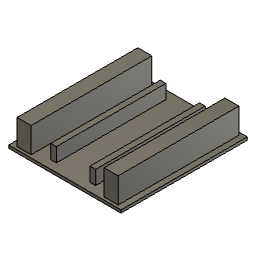
Nano Grove Shield (Autodesk Fusion 360 design; units mm, degrees)
Autodesk Fusion 360 part; units mm, degrees
sketch "Sketch1" plane through (0, 0, 0) normal (0, 1, 0) x (1, 0, 0)
  line L0 (0, 0) -> (40, 0)
  line L1 (40, 0) -> (40, -45)
  line L2 (40, -45) -> (0, -45)
  line L3 (0, -45) -> (0, 0)
  dimension "d1" = 40
  dimension "d2" = 45
  constraint horizontal L0
  constraint vertical L1
  constraint horizontal L2
  constraint vertical L3
  constraint coincident L0.start L3.end
  measures "d1" distance of L0.start L0.end
  measures "d2" distance of L0.start L2.end
extrude "Extrude1" add sketch "Sketch1" along normal blind 1
sketch "Sketch2" plane through (0, 1, 0) normal (0, 1, 0) x (-1, 0, 0)
  line L0 (0, 45) -> (-40, 45)
  line L1 (-40, 45) -> (-40, 0)
  line L2 (-40, 0) -> (0, 0)
  line L3 (0, 0) -> (0, 45)
  line L4 (-2, 1) -> (-7, 1)
  line L5 (-7, 1) -> (-7, 44)
  line L6 (-7, 44) -> (-2, 44)
  line L7 (-2, 44) -> (-2, 1)
  dimension "d5" = 5
  dimension "d6" = 43
  dimension "d7" = 1
  dimension "d8" = 2
  dimension "d9" = 1
  constraint horizontal L4
  constraint vertical L5
  constraint horizontal L6
  constraint vertical L7
  measures "d5" distance of L4.start L4.end
  measures "d6" distance of L4.start L6.end
  measures "d7" distance of L2 L4
  measures "d8" distance of L3 L7
  measures "d9" distance of L0 L6
extrude "Extrude2" add sketch "Sketch2" along normal blind 9 contours L4 L5 L6 L7
sketch "Sketch3" plane through (0, 1, 0) normal (0, 1, 0) x (-1, 0, 0)
  line L0 (-2, 44) -> (-2, 1)
  line L1 (-2, 1) -> (-7, 1)
  line L2 (-7, 1) -> (-7, 44)
  line L3 (-7, 44) -> (-2, 44)
  line L4 (0, 45) -> (-40, 45)
  line L5 (-40, 45) -> (-40, 0)
  line L6 (-40, 0) -> (0, 0)
  line L7 (0, 0) -> (0, 45)
  line L8 (-12, 3) -> (-14, 3)
  line L9 (-14, 3) -> (-14, 42)
  line L10 (-14, 42) -> (-12, 42)
  line L11 (-12, 42) -> (-12, 3)
  dimension "d12" = 2
  dimension "d13" = 39
  dimension "d14" = 5
  dimension "d16" = 3
  dimension "d17" = 3
  constraint horizontal L8
  constraint vertical L9
  constraint horizontal L10
  constraint vertical L11
  measures "d12" distance of L8.start L8.end
  measures "d13" distance of L8.start L10.end
  measures "d14" distance of L2 L11
  measures "d16" distance of L6 L8
  measures "d17" distance of L4 L10
extrude "Extrude3" add sketch "Sketch3" along normal blind 5 contours L8 L9 L10 L11
move_body "Align1" bodies 1 to x (1, 0, 0) y (0, 1, 0) z (0, 0, 1) at (-20, 0, -22.5)
sketch "Sketch5" plane through (0, 1, 0) normal (0, 1, 0) x (-1, 0, 0)
  line L0 (8, 19.5) -> (8, -19.5)
  line L1 (8, -19.5) -> (6, -19.5)
  line L2 (6, -19.5) -> (6, 19.5)
  line L3 (6, 19.5) -> (8, 19.5)
  line L4 (18, 21.5) -> (18, -21.5)
  line L5 (18, -21.5) -> (13, -21.5)
  line L6 (13, -21.5) -> (13, 21.5)
  line L7 (13, 21.5) -> (18, 21.5)
  line L8 (20, 22.5) -> (-20, 22.5)
  line L9 (-20, 22.5) -> (-20, -22.5)
  line L10 (-20, -22.5) -> (20, -22.5)
  line L11 (20, -22.5) -> (20, 22.5)
  line L12 (-13, -21.5) -> (-18, -21.5)
  line L13 (-18, -21.5) -> (-18, 21.5)
  line L14 (-18, 21.5) -> (-13, 21.5)
  line L15 (-13, 21.5) -> (-13, -21.5)
  dimension "d26" = 5
  dimension "d27" = 43
  dimension "d28" = 1
  dimension "d29" = 1
  dimension "d30" = 2
  constraint horizontal L12
  constraint vertical L13
  constraint horizontal L14
  constraint vertical L15
  measures "d26" distance of L12.start L12.end
  measures "d27" distance of L12.start L14.end
  measures "d28" distance of L10 L12
  measures "d29" distance of L8 L14
  measures "d30" distance of L9 L13
extrude "Extrude5" add sketch "Sketch5" along normal blind 9 contours L12 L13 L14 L15
sketch "Sketch6" plane through (0, 1, 0) normal (0, 1, 0) x (-1, 0, 0)
  line L0 (-13, 21.5) -> (-13, -21.5)
  line L1 (-13, -21.5) -> (-18, -21.5)
  line L2 (-18, -21.5) -> (-18, 21.5)
  line L3 (-18, 21.5) -> (-13, 21.5)
  line L4 (8, 19.5) -> (8, -19.5)
  line L5 (8, -19.5) -> (6, -19.5)
  line L6 (6, -19.5) -> (6, 19.5)
  line L7 (6, 19.5) -> (8, 19.5)
  line L8 (18, 21.5) -> (18, -21.5)
  line L9 (18, -21.5) -> (13, -21.5)
  line L10 (13, -21.5) -> (13, 21.5)
  line L11 (13, 21.5) -> (18, 21.5)
  line L12 (20, 22.5) -> (-20, 22.5)
  line L13 (-20, 22.5) -> (-20, -22.5)
  line L14 (-20, -22.5) -> (20, -22.5)
  line L15 (20, -22.5) -> (20, 22.5)
  line L16 (-6, -19.5) -> (-8, -19.5)
  line L17 (-8, -19.5) -> (-8, 19.5)
  line L18 (-8, 19.5) -> (-6, 19.5)
  line L19 (-6, 19.5) -> (-6, -19.5)
  dimension "d33" = 2
  dimension "d34" = 39
  dimension "d35" = 3
  dimension "d36" = 3
  dimension "d37" = 5
  constraint horizontal L16
  constraint vertical L17
  constraint horizontal L18
  constraint vertical L19
  measures "d33" distance of L16.start L16.end
  measures "d34" distance of L16.start L18.end
  measures "d35" distance of L14 L16
  measures "d36" distance of L12 L18
  measures "d37" distance of L0 L17
extrude "Extrude6" add sketch "Sketch6" along normal blind 5 contours L16 L17 L18 L19
